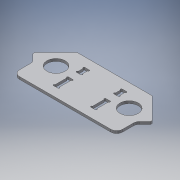
# Autodesk Inventor part: 胴体_メインフレーム_1_1
Saved by Autodesk Inventor 2018 (Build 220112000, 112)
## iProperties
Created: 2016-05-05
Part Number: 胴体_メインフレーム_1_1
Material: アルミニウム 2014-T4
Document SubType Name: Modeling
Designer: hiroaki
Density: 2.8 g/cm^3
Appearance: サテン
Mass: 25.5647 g
Surface Area: 104.556 cm^2
Volume: 9.13025 cm^3
Author: hiroaki
Autodesk Inventor part; units mm, degrees
ref_plane "YZ Plane" through (0, 0, 0) normal (1, 0, 0) x (0, 1, 0)
ref_plane "XZ Plane" through (0, 0, 0) normal (0, 1, 0) x (-1, 0, 0)
ref_plane "XY Plane" through (0, 0, 0) normal (0, 0, 1) x (1, 0, 0)
derived "胴体_基礎_1_1.ipt"
sketch "スケッチ1" plane through (0, 0, 0) normal (0, 0, 1) x (1, 0, 0)
  circle A0 centre (44, 0) radius 10.5 construction
  line L0 (0, 0) -> (0, 13.5711) construction
  line L1 (0, 0) -> (44, 0) construction
  line L2 (30.5, -1) -> (57.5, -1) construction
  line L3 (57.5, -1) -> (57.5, -28) construction
  line L4 (57.5, -28) -> (30.5, -28) construction
  line L5 (30.5, -28) -> (30.5, -1) construction
  circle A1 centre (30.5, -1) radius 1.35
  circle A2 centre (57.5, -1) radius 1.35
  circle A3 centre (30.5, -28) radius 1.35
  circle A4 centre (57.5, -28) radius 1.35
  line L6 (28, 0) -> (28, -39.5) construction
  line L7 (28, -39.5) -> (60, -39.5) construction
  line L8 (60, -39.5) -> (60, 0) construction
  line L9 (44, 0) -> (44, -1) construction
  arc A5 (33.417, 12) -> (28, 0) centre (44, 0) ccw construction
  line L10 (33.417, 12) -> (54.583, 12) construction
  arc A6 (60, 0) -> (54.583, 12) centre (44, 0) ccw construction
  circle A7 centre (44, 0) radius 11
  line L11 (56.5, 21.6506) -> (8, -62.3538) construction
  line L12 (31.8157, -76.1038) -> (-15.8157, -48.6038) construction
  line L13 (-15.8157, -48.6038) -> (32.6843, 35.4006) construction
  line L14 (32.6843, 35.4006) -> (80.3157, 7.9006) construction
  line L15 (80.3157, 7.9006) -> (31.8157, -76.1038) construction
  line L16 (-71.5, 25) -> (-16.5, 25) construction
  line L17 (-16.5, 25) -> (-16.5, -72) construction
  line L18 (-16.5, -72) -> (-71.5, -72) construction
  line L19 (-71.5, -72) -> (-71.5, 25) construction
  line L20 (-44, 25) -> (-44, -72) construction
  line L21 (-71.5, 0) -> (-16.5, 0) construction
  line L22 (-52.5, -44.5) -> (52.5, -44.5) construction
  line L23 (52.5, -44.5) -> (52.5, -78) construction
  line L24 (52.5, -78) -> (-52.5, -78) construction
  line L25 (-52.5, -78) -> (-52.5, -44.5) construction
  line L26 (-44.5, -5) -> (44.5, -5) construction
  line L27 (44.5, -5) -> (44.5, -65) construction
  line L28 (44.5, -65) -> (-44.5, -65) construction
  line L29 (-44.5, -65) -> (-44.5, -5) construction
  circle A8 centre (44, 24.25) radius 1.2
  circle A9 centre (19.75, 0) radius 1.2
  circle A10 centre (44, -24.25) radius 1.2
  circle A11 centre (68.25, 0) radius 1.2
  line L30 (-45.0355, 26.75) -> (45.0355, 26.75)
  circle A12 centre (44, 24.25) radius 2.5 construction
  line L31 (46, 25.4047) -> (46, 23.0953) construction
  line L32 (46, 23.0953) -> (44, 21.9406) construction
  line L33 (44, 21.9406) -> (42, 23.0953) construction
  line L34 (42, 23.0953) -> (42, 25.4047) construction
  line L35 (42, 25.4047) -> (44, 26.5594) construction
  line L36 (44, 26.5594) -> (46, 25.4047) construction
  line L37 (70.75, 1.0355) -> (70.75, -31.2817) construction
  line L38 (-70.75, -31.2817) -> (-70.75, 1.0355) construction
  circle A13 centre (68.25, 0) radius 2.5 construction
  circle A14 centre (-44, 24.25) radius 1.2
  circle A15 centre (-19.75, 0) radius 1.2
  circle A16 centre (-30.5, -1) radius 1.35
  circle A17 centre (-44, 0) radius 11
  circle A18 centre (-57.5, -1) radius 1.35
  circle A19 centre (-44, -24.25) radius 1.2
  circle A20 centre (-30.5, -28) radius 1.35
  circle A21 centre (-57.5, -28) radius 1.35
  circle A22 centre (-68.25, 0) radius 1.2
  line L39 (-45.0355, 26.75) -> (-70.75, 1.0355)
  line L40 (45.0355, 26.75) -> (70.75, 1.0355)
  line L41 (70.75, 1.0355) -> (70.75, -1.0355)
  line L42 (-70.75, 1.0355) -> (-70.75, -1.0355)
  line L43 (-70.75, -1.0355) -> (-62, -9.7855)
  line L44 (-62, -9.7855) -> (-62, -33)
  line L45 (-62, -33) -> (62, -33)
  line L46 (62, -33) -> (62, -9.7855)
  line L47 (62, -9.7855) -> (70.75, -1.0355)
  line L48 (21.5, -5) -> (26.5, -5) construction
  line L49 (19.75, 0) -> (28, 0) construction
  circle A23 centre (22.5, -28) radius 1.55
  circle A24 centre (22.5, 21.75) radius 1.55
  circle A25 centre (-22.5, 21.75) radius 1.55
  circle A26 centre (-22.5, -28) radius 1.55
  circle A27 centre (19.75, 0) radius 2 construction
  circle A28 centre (22.5, 21.75) radius 3 construction
  line L50 (-25.05, 15.75) -> (-19.95, 15.75) construction
  line L51 (-19.95, 15.75) -> (-19.95, 5.75) construction
  line L52 (-19.95, 5.75) -> (-25.05, 5.75) construction
  line L53 (-25.05, 5.75) -> (-25.05, 15.75) construction
  line L54 (-25.05, -4) -> (-19.95, -4) construction
  line L55 (-19.95, -4) -> (-19.95, -22) construction
  line L56 (-19.95, -22) -> (-25.05, -22) construction
  line L57 (-25.05, -22) -> (-25.05, -4) construction
  circle A29 centre (-19.75, 0) radius 2.5 construction
  line L58 (-19.9, 15.8) -> (-25.1, 15.8)
  line L59 (-25.1, 15.8) -> (-25.1, 5.7)
  line L60 (-25.1, 5.7) -> (-19.9, 5.7)
  line L61 (-19.9, 5.7) -> (-19.9, 15.8)
  circle A30 centre (-25.1, 14.75) radius 1.05
  circle A31 centre (-19.9, 14.75) radius 1.05
  circle A32 centre (-19.9, 6.75) radius 1.05
  circle A33 centre (-25.1, 6.75) radius 1.05
  line L62 (-19.9, -3.95) -> (-25.1, -3.95)
  line L63 (-25.1, -3.95) -> (-25.1, -22.05)
  line L64 (-25.1, -22.05) -> (-19.9, -22.05)
  line L65 (-19.9, -22.05) -> (-19.9, -3.95)
  circle A34 centre (-25.1, -5) radius 1.05
  circle A35 centre (-19.9, -5) radius 1.05
  circle A36 centre (-25.1, -21) radius 1.05
  circle A37 centre (-19.9, -21) radius 1.05
  line L66 (25.1, 15.8) -> (25.1, 5.7)
  circle A38 centre (25.1, 14.75) radius 1.05
  line L67 (19.9, 15.8) -> (25.1, 15.8)
  circle A39 centre (19.9, 14.75) radius 1.05
  line L68 (19.9, 5.7) -> (19.9, 15.8)
  circle A40 centre (25.1, 6.75) radius 1.05
  circle A41 centre (19.9, 6.75) radius 1.05
  line L69 (25.1, 5.7) -> (19.9, 5.7)
  circle A42 centre (25.1, -5) radius 1.05
  circle A43 centre (19.9, -5) radius 1.05
  line L70 (19.9, -3.95) -> (25.1, -3.95)
  line L71 (19.9, -22.05) -> (19.9, -3.95)
  line L72 (25.1, -3.95) -> (25.1, -22.05)
  circle A44 centre (25.1, -21) radius 1.05
  circle A45 centre (19.9, -21) radius 1.05
  line L73 (25.1, -22.05) -> (19.9, -22.05)
  circle A46 centre (-68.25, 0) radius 1.2
  circle A47 centre (-44, -24.25) radius 1.2
  circle A48 centre (-19.75, 0) radius 1.2
  circle A49 centre (-44, 24.25) radius 1.2
  circle A50 centre (44, -24.25) radius 1.2
  circle A51 centre (68.25, 0) radius 1.2
  circle A52 centre (44, 24.25) radius 1.2
  circle A53 centre (19.75, 0) radius 1.2
  circle A54 centre (44, 0) radius 21.9406 construction
  point P0 (0, -44.5)
  point P1 (-44.5, -35)
  point P2 (0, -5)
  point P3 (-22.5, 15.75)
  point P4 (-22.5, -4)
  point P5 (-22.5, 5.75)
  dimension "d78" = 2.4
  dimension "d81" = 360
  dimension "d85" = 360
  measures "d78" diameter of A46
extrude "押し出し1" add sketch "スケッチ1" along normal blind 3
fillet "フィレット2" radius 7 4 edges at (62, -33, 1.5) (-62, -33, 1.5) (-62, -9.7855, 1.5) (62, -9.7855, 1.5)
sketch "スケッチ7" plane through (45.0355, 26.75, 0) normal (0, 0, -1) x (-1, 0, 0)
  circle A0 centre (67.5355, -54.75) radius 1.55 projected
  circle A1 centre (67.5355, -54.75) radius 1.55
  circle A2 centre (75.5355, -54.75) radius 1.35 projected
  circle A3 centre (75.5355, -54.75) radius 1.35
  circle A4 centre (89.0355, -51) radius 1.2 projected
  circle A5 centre (89.0355, -51) radius 1.2
  circle A6 centre (102.5355, -54.75) radius 1.35 projected
  circle A7 centre (102.5355, -54.75) radius 1.35
  circle A8 centre (102.5355, -27.75) radius 1.35 projected
  circle A9 centre (102.5355, -27.75) radius 1.35
  circle A10 centre (113.2855, -26.75) radius 1.2 projected
  circle A11 centre (113.2855, -26.75) radius 1.2
  circle A12 centre (75.5355, -27.75) radius 1.35 projected
  circle A13 centre (75.5355, -27.75) radius 1.35
  circle A14 centre (64.7855, -26.75) radius 1.2 projected
  circle A15 centre (64.7855, -26.75) radius 1.2
  circle A16 centre (67.5355, -5) radius 1.55 projected
  circle A17 centre (67.5355, -5) radius 1.55
  circle A18 centre (89.0355, -2.5) radius 1.2 projected
  circle A19 centre (89.0355, -2.5) radius 1.2
  circle A20 centre (25.2855, -26.75) radius 1.2 projected
  circle A21 centre (25.2855, -26.75) radius 1.2
  circle A22 centre (14.5355, -27.75) radius 1.35 projected
  circle A23 centre (14.5355, -27.75) radius 1.35
  circle A24 centre (22.5355, -54.75) radius 1.55 projected
  circle A25 centre (22.5355, -54.75) radius 1.55
  circle A26 centre (14.5355, -54.75) radius 1.35 projected
  circle A27 centre (14.5355, -54.75) radius 1.35
  circle A28 centre (1.0355, -51) radius 1.2 projected
  circle A29 centre (1.0355, -51) radius 1.2
  circle A30 centre (22.5355, -5) radius 1.55 projected
  circle A31 centre (22.5355, -5) radius 1.55
  circle A32 centre (1.0355, -2.5) radius 1.2 projected
  circle A33 centre (1.0355, -2.5) radius 1.2
  circle A34 centre (-12.4645, -27.75) radius 1.35 projected
  circle A35 centre (-12.4645, -27.75) radius 1.35
  circle A36 centre (-23.2145, -26.75) radius 1.2 projected
  circle A37 centre (-23.2145, -26.75) radius 1.2
  circle A38 centre (-12.4645, -54.75) radius 1.35 projected
  circle A39 centre (-12.4645, -54.75) radius 1.35
  point P0 (45.0355, -26.75)
  constraints: 20 centre point, 20 coincident
extrude "押し出し4" add sketch "スケッチ7" against normal up to surface (3 mm away)
equation "\"d48\" = 3"
